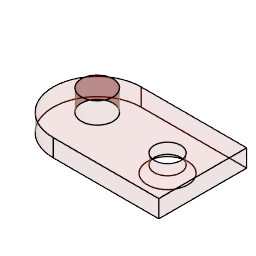
verdure-buddy (Autodesk Fusion 360 archive; units mm, degrees)
design "导光柱"
Autodesk Fusion 360 part; units mm, degrees
sketch "草图1" plane through (0, 0, 0) normal (0, 1, 0) x (1, 0, 0)
  line L0 (4.25, -2.5) -> (-4.25, -2.5)
  line L1 (-4.25, -2.5) -> (-4.25, 2.5)
  line L2 (-4.25, 2.5) -> (4.25, 2.5)
  line L3 (4.25, 2.5) -> (4.25, -2.5)
  line L4 (4.25, -2.5) -> (-4.25, 2.5) construction
  line L5 (-4.25, -2.5) -> (4.25, 2.5) construction
  dimension "d1" = 8.5
  dimension "d2" = 5
  constraint horizontal L0
  constraint perpendicular L0 L1
  constraint parallel L0 L2
  constraint parallel L1 L3
  constraint coincident L4 origin
  constraint coincident L5 origin
  measures "d1" distance of L1.end L2.end
  measures "d2" distance of L0.end L1.end
extrude "拉伸1" add sketch "草图1" along normal blind 1
sketch "草图2" plane through (0, 1, 0) normal (0, 1, 0) x (-1, 0, 0)
  line L0 (-4.25, -2.5) -> (4.25, -2.5)
  line L1 (4.25, -2.5) -> (4.25, 2.5)
  line L2 (4.25, 2.5) -> (-4.25, 2.5)
  line L3 (-4.25, 2.5) -> (-4.25, -2.5)
  circle A0 centre (-2.25, 0) radius 0.75
  circle A1 centre (1.75, 0) radius 0.9
  dimension "d5" = 1.5
  dimension "d6" = 2
  dimension "d7" = 1.8
  dimension "d8" = 4
  measures "d5" diameter of A0
  measures "d6" distance of L3 A0.centre
  measures "d7" diameter of A1
  measures "d8" distance of A0.centre A1.centre
extrude "拉伸2" add sketch "草图2" along normal blind 1.2 contours A1
extrude "拉伸3" cut sketch "草图2" against normal blind 3.5 contours A0
chamfer "倒角1" distance 0.4 angle 45 1 edges at (2.9492, 0, -0.2712)
fillet "圆角1" radius 2.5 2 edges at (-4.25, 0.5, 2.5) (-4.25, 0.5, -2.5)
